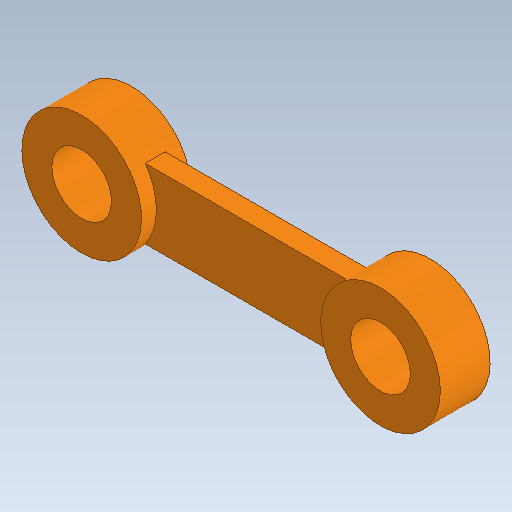
# Autodesk Inventor part: Conrod
Saved by Autodesk Inventor 2020.5 (Build 245400000, 400)
## iProperties
Created: 2018-04-07
Part Number: Conrod
Document SubType Name: Modeling
Designer: Administrator
Density: 7.85 g/cm^3
Mass: 8.71598 g
Surface Area: 12.1798 cm^2
Volume: 1.11032 cm^3
Material: Acero, carbono
Appearance: Orange
Author: Administrator
Autodesk Inventor part; units mm, degrees
ref_plane "YZ Plane" through (0, 0, 0) normal (1, 0, 0) x (0, 1, 0)
ref_plane "XZ Plane" through (0, 0, 0) normal (0, 1, 0) x (-1, 0, 0)
ref_plane "XY Plane" through (0, 0, 0) normal (0, 0, 1) x (1, 0, 0)
sketch "Sketch1" plane through (0, 0, 0) normal (0, 0, 1) x (1, 0, 0)
  line L0 (0, 0) -> (30, 0)
  circle A0 centre (0, 0) radius 3
  circle A1 centre (30, 0) radius 3
  circle A2 centre (0, 0) radius 6
  circle A3 centre (30, 0) radius 6
  line L1 (4.8734, 3.5) -> (25.1266, 3.5)
  line L2 (4.8734, -3.5) -> (25.1266, -3.5)
  dimension "d0" = 30
  dimension "d1" = 6
  dimension "d2" = 12
  dimension "d3" = 7
  constraints: 6 end point, 4 centre point, 4 coincident, 4 point on circle, 3 parallel, 2 equal radius, 1 horizontal, 1 other
  measures "d0" distance of L0.start L0.end
  measures "d1" diameter of A0
  measures "d2" diameter of A2
  measures "d3" distance between parallel lines of L1 L2
extrude "Extrusion1" add sketch "Sketch1" along normal mid plane 5
sketch "Sketch2" plane through (0, 0, 2.5) normal (0, 0, 1) x (1, 0, 0)
  arc A0 (25.1266, -3.5) -> (25.1266, 3.5) centre (30, 0) ccw projected
  line L0 (4.8734, 3.5) -> (25.1266, 3.5) projected
  arc A1 (4.8734, 3.5) -> (4.8734, -3.5) centre (0, 0) ccw projected
  line L1 (25.1266, -3.5) -> (4.8734, -3.5) projected
  circle A2 centre (0, 0) radius 6
  circle A3 centre (30, 0) radius 6
  constraints: 2 centre point, 2 coincident, 2 concentric
extrude "Extrusion2" cut sketch "Sketch2" against normal blind 1.5 contours L1 A2 L0 A3
mirror "Mirror1" about plane through (0, 0, 0) normal (0, 0, 1) of "Extrusion2"
body "Solid1"
